Autodesk Fusion 360 part; units mm, degrees
(part 4 of 4)
  arc A34 (58.0734, 20.2895) -> (58.0734, 21.7816) centre (42.8517, 21.0355) ccw
  spline S17 degree 5 poles (54.6097, 23.0779) (54.6197, 23.0796) (54.6395, 23.0827) (54.6694, 23.0863) (54.7095, 23.0891) (54.7598, 23.09) (54.8103, 23.0889) (54.8609, 23.0867) (54.9115, 23.0838) (54.9622, 23.0806) (55.0129, 23.0768) (55.0636, 23.0724) (55.1143, 23.0671) (55.1651, 23.0609) (55.216, 23.0537) (55.2668, 23.0456) (55.3176, 23.0368) (55.3685, 23.0274) (55.4193, 23.0175) (55.4701, 23.007) (55.5209, 22.996) (55.5717, 22.9844) (55.6224, 22.9723) (55.6731, 22.9595) (55.7238, 22.9461) (55.7745, 22.9322) (55.8251, 22.9177) (55.8757, 22.9027) (55.9262, 22.8873) (55.9767, 22.8713) (56.0271, 22.8548) (56.0775, 22.8379) (56.1278, 22.8205) (56.1781, 22.8026) (56.2283, 22.7842) (56.2785, 22.7653) (56.3286, 22.746) (56.3786, 22.7263) (56.4286, 22.7061) (56.4785, 22.6854) (56.5283, 22.6644) (56.578, 22.6429) (56.6277, 22.6209) (56.6773, 22.5986) (56.7268, 22.5758) (56.7762, 22.5526) (56.8256, 22.529) (56.8748, 22.505) (56.924, 22.4806) (56.9731, 22.4557) (57.0221, 22.4305) (57.071, 22.4049) (57.1198, 22.3789) (57.1685, 22.3526) (57.2171, 22.3258) (57.2656, 22.2987) (57.314, 22.2711) (57.3623, 22.2432) (57.4105, 22.215) (57.4586, 22.1863) (57.5066, 22.1573) (57.5545, 22.128) (57.6022, 22.0982) (57.6499, 22.0682) (57.6974, 22.0377) (57.7448, 22.0069) (57.7922, 21.9758) (57.8393, 21.9443) (57.8864, 21.9125) (57.9334, 21.8803) (57.9802, 21.8478) (58.0175, 21.8215) (58.0455, 21.8016) (58.0641, 21.7883) (58.0734, 21.7816) knots 0 0 0 0 0 0 0.01428571 0.02857143 0.04285714 0.05714286 0.07142857 0.08571429 0.1 0.11428571 0.12857143 0.14285714 0.15714286 0.17142857 0.18571429 0.2 0.21428571 0.22857143 0.24285714 0.25714286 0.27142857 0.28571429 0.3 0.31428571 0.32857143 0.34285714 0.35714286 0.37142857 0.38571429 0.4 0.41428571 0.42857143 0.44285714 0.45714286 0.47142857 0.48571429 0.5 0.51428571 0.52857143 0.54285714 0.55714286 0.57142857 0.58571429 0.6 0.61428571 0.62857143 0.64285714 0.65714286 0.67142857 0.68571429 0.7 0.71428571 0.72857143 0.74285714 0.75714286 0.77142857 0.78571429 0.8 0.81428571 0.82857143 0.84285714 0.85714286 0.87142857 0.88571429 0.9 0.91428571 0.92857143 0.94285714 0.95714286 0.97142857 0.98571429 1 1 1 1 1 1
  line L17 (54.6097, 23.0779) -> (52.659, 22.7394)
  arc A35 (52.2938, 22.9879) -> (52.659, 22.7394) centre (52.6047, 23.0522) ccw
  arc A36 (52.2938, 22.9879) -> (51.6381, 25.006) centre (42.8517, 21.0355) ccw
  arc A37 (51.7875, 25.4217) -> (51.6381, 25.006) centre (51.9274, 25.1367) ccw
  line L18 (51.7875, 25.4217) -> (53.5646, 26.2944)
  spline S18 degree 5 poles (53.5646, 26.2944) (53.5737, 26.2989) (53.5916, 26.308) (53.6179, 26.3227) (53.6519, 26.344) (53.6931, 26.3729) (53.7333, 26.4034) (53.7729, 26.435) (53.8123, 26.467) (53.8513, 26.4994) (53.8901, 26.5323) (53.9286, 26.5657) (53.9665, 26.5998) (54.0039, 26.6347) (54.0408, 26.6704) (54.0772, 26.7068) (54.1132, 26.7438) (54.1488, 26.7812) (54.1841, 26.8192) (54.219, 26.8575) (54.2536, 26.8962) (54.2879, 26.9355) (54.3218, 26.9751) (54.3553, 27.0153) (54.3885, 27.0559) (54.4212, 27.0969) (54.4537, 27.1384) (54.4858, 27.1803) (54.5176, 27.2225) (54.5491, 27.2651) (54.5802, 27.308) (54.611, 27.3513) (54.6415, 27.395) (54.6716, 27.4391) (54.7015, 27.4834) (54.731, 27.5282) (54.7601, 27.5732) (54.789, 27.6186) (54.8175, 27.6643) (54.8458, 27.7104) (54.8737, 27.7567) (54.9013, 27.8033) (54.9286, 27.8503) (54.9556, 27.8975) (54.9822, 27.945) (55.0086, 27.9929) (55.0346, 28.041) (55.0604, 28.0893) (55.0858, 28.138) (55.1109, 28.1869) (55.1357, 28.2361) (55.1602, 28.2856) (55.1844, 28.3353) (55.2083, 28.3853) (55.2319, 28.4355) (55.2552, 28.486) (55.2782, 28.5367) (55.3009, 28.5876) (55.3233, 28.6388) (55.3454, 28.6903) (55.3671, 28.7419) (55.3886, 28.7938) (55.4098, 28.8459) (55.4306, 28.8983) (55.4512, 28.9509) (55.4715, 29.0036) (55.4914, 29.0566) (55.5111, 29.1099) (55.5305, 29.1633) (55.5495, 29.2169) (55.5683, 29.2707) (55.5831, 29.314) (55.594, 29.3465) (55.6013, 29.3682) (55.6049, 29.379) knots 0 0 0 0 0 0 0.01428571 0.02857143 0.04285714 0.05714286 0.07142857 0.08571429 0.1 0.11428571 0.12857143 0.14285714 0.15714286 0.17142857 0.18571429 0.2 0.21428571 0.22857143 0.24285714 0.25714286 0.27142857 0.28571429 0.3 0.31428571 0.32857143 0.34285714 0.35714286 0.37142857 0.38571429 0.4 0.41428571 0.42857143 0.44285714 0.45714286 0.47142857 0.48571429 0.5 0.51428571 0.52857143 0.54285714 0.55714286 0.57142857 0.58571429 0.6 0.61428571 0.62857143 0.64285714 0.65714286 0.67142857 0.68571429 0.7 0.71428571 0.72857143 0.74285714 0.75714286 0.77142857 0.78571429 0.8 0.81428571 0.82857143 0.84285714 0.85714286 0.87142857 0.88571429 0.9 0.91428571 0.92857143 0.94285714 0.95714286 0.97142857 0.98571429 1 1 1 1 1 1
  arc A38 (55.6049, 29.379) -> (54.7278, 30.5863) centre (42.8517, 21.0355) ccw
  spline S19 degree 5 poles (51.1637, 29.5991) (51.1707, 29.6063) (51.1849, 29.6205) (51.207, 29.6409) (51.2378, 29.6668) (51.278, 29.697) (51.3195, 29.7258) (51.3617, 29.7538) (51.4043, 29.7812) (51.4472, 29.8084) (51.4905, 29.8351) (51.5341, 29.8614) (51.5783, 29.8869) (51.623, 29.9117) (51.6684, 29.9358) (51.7142, 29.9591) (51.7605, 29.9819) (51.8072, 30.0042) (51.8541, 30.026) (51.9014, 30.0474) (51.9489, 30.0684) (51.9968, 30.0888) (52.045, 30.1088) (52.0936, 30.1283) (52.1424, 30.1473) (52.1916, 30.1658) (52.2411, 30.1838) (52.2908, 30.2014) (52.3408, 30.2186) (52.391, 30.2354) (52.4415, 30.2517) (52.4922, 30.2676) (52.5432, 30.2831) (52.5944, 30.2982) (52.6458, 30.3128) (52.6975, 30.3271) (52.7493, 30.3409) (52.8014, 30.3543) (52.8537, 30.3673) (52.9062, 30.38) (52.9589, 30.3922) (53.0118, 30.404) (53.0649, 30.4155) (53.1181, 30.4265) (53.1716, 30.4372) (53.2252, 30.4475) (53.279, 30.4574) (53.3329, 30.4669) (53.3871, 30.4761) (53.4414, 30.4849) (53.4958, 30.4933) (53.5504, 30.5013) (53.6052, 30.5089) (53.6601, 30.5162) (53.7152, 30.5231) (53.7704, 30.5297) (53.8257, 30.5359) (53.8812, 30.5417) (53.9368, 30.5472) (53.9925, 30.5523) (54.0484, 30.557) (54.1044, 30.5614) (54.1605, 30.5654) (54.2167, 30.5691) (54.2731, 30.5724) (54.3295, 30.5754) (54.3861, 30.578) (54.4428, 30.5803) (54.4996, 30.5822) (54.5565, 30.5837) (54.6135, 30.585) (54.6591, 30.5857) (54.6935, 30.586) (54.7163, 30.5862) (54.7278, 30.5863) knots 0 0 0 0 0 0 0.01428571 0.02857143 0.04285714 0.05714286 0.07142857 0.08571429 0.1 0.11428571 0.12857143 0.14285714 0.15714286 0.17142857 0.18571429 0.2 0.21428571 0.22857143 0.24285714 0.25714286 0.27142857 0.28571429 0.3 0.31428571 0.32857143 0.34285714 0.35714286 0.37142857 0.38571429 0.4 0.41428571 0.42857143 0.44285714 0.45714286 0.47142857 0.48571429 0.5 0.51428571 0.52857143 0.54285714 0.55714286 0.57142857 0.58571429 0.6 0.61428571 0.62857143 0.64285714 0.65714286 0.67142857 0.68571429 0.7 0.71428571 0.72857143 0.74285714 0.75714286 0.77142857 0.78571429 0.8 0.81428571 0.82857143 0.84285714 0.85714286 0.87142857 0.88571429 0.9 0.91428571 0.92857143 0.94285714 0.95714286 0.97142857 0.98571429 1 1 1 1 1 1
  line L19 (51.1637, 29.5991) -> (49.7845, 28.1786)
  arc A39 (49.343, 28.165) -> (49.7845, 28.1786) centre (49.5567, 28.3997) ccw
  arc A40 (49.343, 28.165) -> (47.6263, 29.4122) centre (42.8517, 21.0355) ccw
  circle A41 centre (42.8517, 21.0355) radius 1.6
  dimension "d30" = 3.2
  constraint concentric A0 A41
  measures "d30" diameter of A41
extrude "Extrude5" cut sketch "Sketch4" against normal blind 5.27 contours A41 in component "Spur Gear (10 teeth)"
component "Spur Gear (10 teeth)" placed x (1, 0, 0) y (0, 1, 0) z (0, 0, 1) at (0, 0, 0)
equation "d24 = -1.27 mm + 10 mm"
